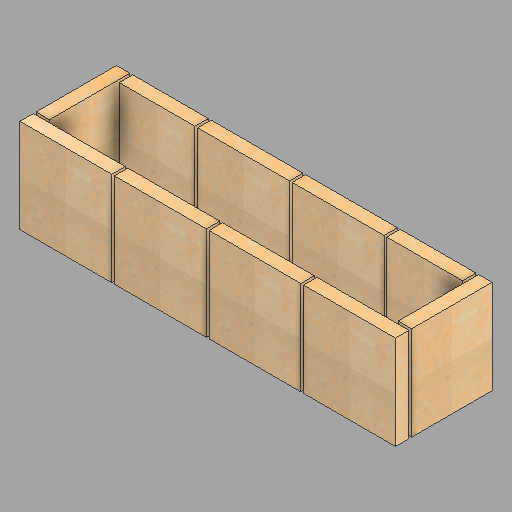
# Autodesk Inventor part: Standard - Amber select
Saved by Autodesk Inventor 2022.2 (Build 262287010, 287A)
## iProperties
Created: 2022-03-28
Part Number: Standard - Amber select
Material: Granite, Cut, Polished
Document SubType Name: Modeling
Designer: awelt
Mass: 311651 g
Surface Area: 47193.5 cm^2
Volume: 115426 cm^3
Density: 2.7 g/cm^3
Appearance: Amber Select
AfterDocSave0: Convert in3 volume to ft3
in3 to ft3: 4.08
TEST: 4.076
Author: awelt
Autodesk Inventor part; units mm, degrees
ref_plane "YZ Plane" through (0, 0, 0) normal (1, 0, 0) x (0, 1, 0)
ref_plane "XZ Plane" through (0, 0, 0) normal (0, 1, 0) x (-1, 0, 0)
ref_plane "XY Plane" through (0, 0, 0) normal (0, 0, 1) x (1, 0, 0)
sketch "Sketch1" plane through (0, 0, 0) normal (0, 0, 1) x (1, 0, 0)
  line L0 (0, 0) -> (1778, 0)
  line L1 (1778, 0) -> (1778, 457.2)
  line L2 (1778, 457.2) -> (0, 457.2)
  line L3 (0, 457.2) -> (0, 0)
  line L4 (434.975, 457.2) -> (434.975, 0)
  line L5 (447.675, 457.2) -> (447.675, 0)
  line L6 (882.65, 457.2) -> (882.65, 0)
  line L7 (895.35, 457.2) -> (895.35, 0)
  line L8 (1330.325, 457.2) -> (1330.325, 0)
  line L9 (1343.025, 457.2) -> (1343.025, 0)
  dimension "d0" = 1778
  dimension "d1" = 457.2
  dimension "d2" = 434.975
  dimension "d3" = 12.7
  dimension "d4" = 434.975
  dimension "d5" = 12.7
  dimension "d6" = 434.975
  dimension "d7" = 12.7
  dimension "d8" = 434.975
  constraints: 20 end point, 8 parallel, 1 horizontal, 1 perpendicular
  measures "d0" distance of L2.end L1.end
  measures "d1" distance of L1.end L0.end
  measures "d2" distance between parallel lines of L3 L4
  measures "d3" distance between parallel lines of L4 L5
  measures "d4" distance between parallel lines of L5 L6
  measures "d5" distance between parallel lines of L6 L7
  measures "d6" distance between parallel lines of L7 L8
  measures "d7" distance between parallel lines of L8 L9
  measures "d8" distance between parallel lines of L1 L9
extrude "Extrusion1" add sketch "Sketch1" along normal blind 63.5 contours L3 L2 L4 L0
extrude "Extrusion2" add sketch "Sketch1" along normal blind 63.5 separate body contours L5 L2 L6 L0
extrude "Extrusion3" add sketch "Sketch1" along normal blind 63.5 separate body contours L7 L2 L8 L0
extrude "Extrusion4" add sketch "Sketch1" along normal blind 63.5 separate body contours L9 L2 L1 L0
sketch "Sketch2" plane through (1778, 0, 0) normal (1, 0, 0) x (0, 0, -1)
  line L0 (0, 0) -> (0, 457.2) projected
  line L1 (12.7, 457.2) -> (12.7, 0)
  line L2 (0, 457.2) -> (-63.5, 457.2) projected
  line L3 (393.7, 457.2) -> (393.7, 0)
  line L4 (393.7, 0) -> (12.7, 0)
  line L5 (-63.5, 457.2) -> (0, 457.2)
  line L6 (12.7, 457.2) -> (393.7, 457.2)
  line L7 (0, 457.2) -> (-63.5, 457.2) projected
  dimension "d17" = 12.7
  dimension "d19" = 381
  dimension "d20" = 457.2
  constraints: 11 end point, 3 collinear, 3 perpendicular, 1 parallel
  measures "d17" distance between parallel lines of L0 L1
  measures "d19" distance between parallel lines of L3 L1
  measures "d20" distance between parallel lines of L4 L6
extrude "Extrusion5" add sketch "Sketch2" against normal blind 63.5 separate body
ref_plane "Work Plane1" through (889, 0, 0) normal (1, 0, 0) x (0, 0, -1)
mirror "Mirror1" about plane through (889, 0, 0) normal (1, 0, 0) bodies 5 separate body
sketch "Sketch3" plane through (1778, 0, -393.7) normal (0, 0, -1) x (-1, 0, 0)
  line L0 (63.5, 457.2) -> (63.5, 0) projected
  line L1 (1714.5, 457.2) -> (1714.5, 0) projected
  line L2 (434.975, 457.2) -> (434.975, 0) projected
  line L3 (447.675, 457.2) -> (447.675, 0) projected
  line L4 (882.65, 457.2) -> (882.65, 0) projected
  line L5 (895.35, 457.2) -> (895.35, 0) projected
  line L6 (1330.325, 457.2) -> (1330.325, 0) projected
  line L7 (1343.025, 457.2) -> (1343.025, 0) projected
  line L8 (0, 457.2) -> (434.975, 457.2) projected
  line L9 (76.2, 457.2) -> (434.975, 457.2)
  line L10 (434.975, 457.2) -> (434.975, 0)
  line L11 (434.975, 0) -> (76.2, 0)
  line L12 (76.2, 0) -> (76.2, 457.2)
  line L13 (447.675, 457.2) -> (882.65, 457.2) projected
  line L14 (447.675, 457.2) -> (882.65, 457.2)
  line L15 (882.65, 457.2) -> (882.65, 0)
  line L16 (882.65, 0) -> (447.675, 0)
  line L17 (447.675, 0) -> (447.675, 457.2)
  line L18 (895.35, 457.2) -> (1330.325, 457.2) projected
  line L19 (1330.325, 0) -> (895.35, 0) projected
  line L20 (895.35, 457.2) -> (1330.325, 457.2)
  line L21 (1330.325, 457.2) -> (1330.325, 0)
  line L22 (1330.325, 0) -> (895.35, 0)
  line L23 (895.35, 0) -> (895.35, 457.2)
  line L24 (1343.025, 457.2) -> (1701.8, 457.2)
  line L25 (1701.8, 457.2) -> (1701.8, 0)
  line L26 (1701.8, 0) -> (1343.025, 0)
  line L27 (1343.025, 0) -> (1343.025, 457.2)
  point P0 (1778, 0)
  dimension "d23" = 12.7
  dimension "d24" = 12.7
  constraints: 32 end point, 8 parallel, 4 horizontal, 4 perpendicular, 2 point on line
  measures "d23" distance between parallel lines of L0 L12
  measures "d24" distance between parallel lines of L25 L1
extrude "Extrusion6" add sketch "Sketch3" against normal blind 63.5 separate body contours L2 L11 L12 L8
extrude "Extrusion7" add sketch "Sketch3" against normal blind 63.5 separate body contours L13 L4 L16 L3
extrude "Extrusion8" add sketch "Sketch3" against normal blind 63.5 separate body contours L18 L6 L19 L5
extrude "Extrusion9" add sketch "Sketch3" against normal blind 63.5 separate body contours L24 L25 L26 L7
move faces "Move1" translate (0, 12.7, 0) faces at (1756.8333, 0, -139.7)
move faces "Move2" translate (0, 12.7, 0) faces at (1582.2083, 0, -351.3667)
move faces "Move3" translate (0, 12.7, 0) faces at (1185.3333, 0, -372.5333)
move faces "Move4" translate (0, 12.7, 0) faces at (737.6583, 0, -372.5333)
move faces "Move5" translate (0, 12.7, 0) faces at (315.3833, 0, -372.5333)
move faces "Move6" translate (0, 12.7, 0) faces at (21.1667, 0, -139.7)
move faces "Move7" translate (0, 12.7, 0) faces at (144.9917, 0, 21.1667)
move faces "Move8" translate (0, 12.7, 0) faces at (592.6667, 0, 21.1667)
move faces "Move9" translate (0, 12.7, 0) faces at (1040.3417, 0, 42.3333)
move faces "Move10" translate (0, 12.7, 0) faces at (1488.0167, 0, 21.1667)
body "Solid1"
body "Solid2"
body "Solid3"
body "Solid4"
body "Solid5"
body "Solid6"
body "Solid7"
body "Solid8"
body "Solid9"
body "Solid10"
